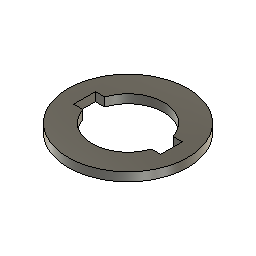
Boat Fuel Tank Gasket (OutD=55) (Autodesk Fusion 360 design; units mm, degrees)
Autodesk Fusion 360 part; units mm, degrees
sketch "Sketch1" plane through (0, 0, 0) normal (0, 0, 1) x (1, 0, 0)
  circle A0 centre (0, 0) radius 27.5
  circle A1 centre (0, 0) radius 16.5
  dimension "d1" = 55
  dimension "d2" = 33
  constraint coincident A0.centre A1.centre
  constraint concentric A0 A1
  measures "d1" diameter of A0
  measures "d2" diameter of A1
extrude "Extrude1" add sketch "Sketch1" along normal blind 4
sketch "Sketch2" plane through (0, 0, 4) normal (0, 0, 1) x (-1, 0, 0)
  circle A0 centre (0, 0) radius 16.5
  circle A1 centre (0, 0) radius 27.5
  line L0 (20, -5) -> (-20, -5)
  line L1 (-20, -5) -> (-20, 5)
  line L2 (-20, 5) -> (20, 5)
  line L3 (20, 5) -> (20, -5)
  constraint horizontal L0
  constraint vertical L1
  constraint horizontal L2
  constraint vertical L3
extrude "Extrude2" cut sketch "Sketch2" against normal blind 15 contours A0 L0 L2 L3 | A0 L0 L1 L2
